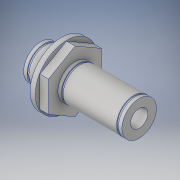
# Autodesk Inventor part: Turret Idle Pin
Saved by Autodesk Inventor 2019.4 (Build 234330000, 330)
## iProperties
Created: 2020-01-23
Part Number: Turret Idle Pin
Material: Aluminum 6061
Document SubType Name: Modeling
Designer: admin
Density: 2.7 g/cm^3
Appearance: Aluminum - Flat
Mass: 49.4424 g
Surface Area: 79.2633 cm^2
Volume: 18.312 cm^3
Author: admin
Autodesk Inventor part; units mm, degrees
ref_plane "YZ Plane" through (0, 0, 0) normal (1, 0, 0) x (0, 1, 0)
ref_plane "XZ Plane" through (0, 0, 0) normal (0, 1, 0) x (-1, 0, 0)
ref_plane "XY Plane" through (0, 0, 0) normal (0, 0, 1) x (1, 0, 0)
sketch "Sketch1" plane through (0, 0, 0) normal (0, 0, 1) x (1, 0, 0)
  line L0 (0, 0) -> (0, 10)
  line L1 (0, 10) -> (2, 10)
  line L2 (2, 10) -> (2, 9.5)
  line L3 (2, 9.5) -> (3.1, 9.5)
  line L4 (3.1, 9.5) -> (3.1, 10)
  line L5 (3.1, 10) -> (11.6, 10)
  line L6 (19.9, 10) -> (21.9, 10)
  line L7 (57.1, 0) -> (0, 0)
  line L8 (21.9, 10) -> (21.9, 9.5)
  line L9 (21.9, 9.5) -> (23, 9.5)
  line L10 (23, 9.5) -> (23, 10)
  line L11 (23, 10) -> (54, 10)
  line L12 (54, 10) -> (54, 9.5)
  line L13 (54, 9.5) -> (55.1, 9.5)
  line L14 (55.1, 9.5) -> (55.1, 10)
  line L15 (55.1, 10) -> (57.1, 10)
  line L16 (57.1, 10) -> (57.1, 0)
  line L17 (19.9, 18) -> (14.9, 18)
  line L18 (14.9, 18) -> (14.9, 18.1)
  line L19 (14.9, 18.1) -> (11.9, 18.1)
  line L20 (11.9, 18.1) -> (11.9, 12)
  line L21 (11.9, 12) -> (11.6, 12)
  line L22 (11.6, 12) -> (11.6, 10)
  line L23 (19.9, 10) -> (19.9, 18)
  dimension "d0" = 1.1
  dimension "d1" = 2
  dimension "d2" = 0.5
  dimension "d8" = 2
  dimension "d9" = 10
  dimension "d18" = 0.5
  dimension "d19" = 1.1
  dimension "d20" = 0.5
  dimension "d21" = 2
  dimension "d22" = 1.1
  dimension "d23" = 31
  dimension "d31" = 18
  dimension "d32" = 3
  dimension "d33" = 0.3
  dimension "d34" = 0.1
  dimension "d35" = 2
  dimension "d36" = 8.5
  dimension "d37" = 5
  dimension "d38" = 10
  constraints: 48 end point, 14 perpendicular, 6 point on line, 4 vertical, 2 horizontal
  measures "d0" distance of L2.end L3.end
  measures "d1" distance of L0.end L1.end
  measures "d2" distance of L1.end L2.end
  measures "d8" distance of L6.start L6.end
  measures "d9" distance between parallel lines of L7 L5
  measures "d18" distance of L6.end L8.end
  measures "d19" distance of L8.end L9.end
  measures "d20" distance of L9.end L10.end
  measures "d21" distance of L14.end L15.end
  measures "d22" distance of L12.end L13.end
  measures "d23" distance of L10.end L11.end
  measures "d31" distance between parallel lines of L7 L17
  measures "d32" distance of L18.end L19.end
  measures "d33" distance of L20.end L21.end
  measures "d34" distance of L17.end L18.end
  measures "d35" distance of L21.end L5.end
  measures "d36" distance of L4.end L5.end
  measures "d37" distance of L17.start L17.end
  measures "d38" distance between parallel lines of L7 L11
revolve "Revolution1" add sketch "Sketch1" angle 360 about axis through (57.1, 0, 0) along (-1, 0, 0)
sketch "Sketch3" plane through (57.1, 0, 0) normal (1, 0, 0) x (0, 0, -1)
  circle A0 centre (0, 0) radius 10 projected
  constraints: 1 coincident
hole "Hole2" at (57.1, 0, 0) direction (-1, 0, 0) diameter 10 end through all
sketch "Sketch4" plane through (19.9, 0, 0) normal (1, 0, 0) x (0, 0, -1)
  line L0 (0, 17.7824) -> (15.4, 8.8912)
  line L1 (15.4, 8.8912) -> (15.4, -8.8912)
  line L2 (15.4, -8.8912) -> (0, -17.7824)
  line L3 (0, -17.7824) -> (-15.4, -8.8912)
  line L4 (-15.4, -8.8912) -> (-15.4, 8.8912)
  line L5 (-15.4, 8.8912) -> (0, 17.7824)
  circle A0 centre (0, 0) radius 18 projected
  dimension "d41" = 30.8
  constraints: 12 end point, 1 coincident, 13 other
  measures "d41" distance between parallel lines of L4 L1
extrude "Extrusion1" cut sketch "Sketch4" against normal up to surface (5 mm away)
body "Solid1"
